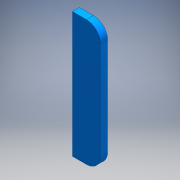
# Autodesk Inventor part: bottomSideFrame
Saved by Autodesk Inventor 2016 (Build 200138000, 138)
## iProperties
Created: 2016-06-05
Part Number: bottomSideFrame
Material: ABS Plastic
Document SubType Name: Modeling
Designer: hesaon
Density: 1.06 g/cm^3
Appearance: Smooth - White
Author: hesaon
Autodesk Inventor part; units mm, degrees
ref_plane "YZ Plane" through (0, 0, 0) normal (1, 0, 0) x (0, 1, 0)
ref_plane "XZ Plane" through (0, 0, 0) normal (0, 1, 0) x (-1, 0, 0)
ref_plane "XY Plane" through (0, 0, 0) normal (0, 0, 1) x (1, 0, 0)
sketch "Sketch1" plane through (0, 0, 0) normal (0, 1, 0) x (-1, 0, 0)
  line L0 (0, 0) -> (-40, 0)
  line L1 (-40, -20) -> (-40, -158)
  line L2 (-20, -178) -> (0, -178)
  line L3 (0, -178) -> (0, 0)
  arc A0 (-20, 0) -> (-40, -20) centre (-20, -20) ccw
  line L4 (-20, -20) -> (-40, -20) construction
  line L5 (-20, -20) -> (-20, 0) construction
  arc A1 (-40, -158) -> (-20, -178) centre (-20, -158) ccw
  line L6 (-20, -158) -> (-20, -178) construction
  line L7 (-20, -158) -> (-40, -158) construction
  dimension "d2" = 90
  dimension "d3" = 20
  dimension "d4" = 20
  dimension "d6" = 90
  dimension "d10" = 20
  dimension "d11" = 20
  dimension "d12" = 178
  constraints: 16 end point, 4 point on circle, 3 parallel, 2 centre point, 1 horizontal, 1 midpoint, 1 perpendicular
  measures "d2" angle of L5 L4
  measures "d3" distance of L5.end L4.start
  measures "d4" horizontal distance of L4.start L0.start
  measures "d6" angle of L7 L6
  measures "d10" horizontal distance of L5.end L1.start
  measures "d11" horizontal distance of L1.end L2.start
  measures "d12" distance of L2.end L0.start
extrude "Extrusion1" add sketch "Sketch1" along normal blind 10
body "Solid1"
